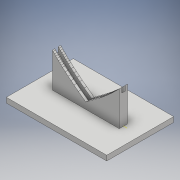
# Autodesk Inventor part: Supporto2
Saved by Autodesk Inventor 2018 (Build 220112000, 112)
## iProperties
Created: 2020-01-19
Part Number: Supporto2
Material: Generic
Document SubType Name: Modeling
Designer: Lorenzo Spadaro
Density: 1 g/cm^3
Appearance: Default
Author: Lorenzo Spadaro
Autodesk Inventor part; units mm, degrees
ref_plane "YZ Plane" through (0, 0, 0) normal (1, 0, 0) x (0, 1, 0)
ref_plane "XZ Plane" through (0, 0, 0) normal (0, 1, 0) x (-1, 0, 0)
ref_plane "XY Plane" through (0, 0, 0) normal (0, 0, 1) x (1, 0, 0)
sketch "Sketch1" plane through (0, 0, 0) normal (0, 0, 1) x (1, 0, 0)
  line L0 (-20, -20) -> (20, -20)
  line L1 (20, -20) -> (20, 20)
  line L2 (20, 20) -> (-20, 20)
  line L3 (-20, 20) -> (-20, -20)
  line L4 (-20, -20) -> (20, 20) construction
  line L5 (20, -20) -> (-20, 20) construction
  point P0 (0, 0)
  dimension "d0" = 40
  dimension "d1" = 40
  constraints: 12 end point, 2 midpoint, 2 parallel, 1 horizontal, 1 perpendicular
  measures "d0" distance of L2.end L1.end
  measures "d1" distance of L1.end L0.end
extrude "Extrusion1" add sketch "Sketch1" along normal blind 3
ref_plane "Work Plane1" through (-20, 0, 0) normal (0, -1, 0) x (1, 0, 0)
sketch "Sketch2" plane through (-20, 0, 0) normal (0, -1, 0) x (1, 0, 0)
  line L0 (0, 3) -> (40, 3)
  line L1 (0, 3) -> (40, 3) projected
  line L2 (2.7399, 64.6358) -> (3.1064, 64.6633)
  line L3 (3.1064, 64.6633) -> (5.3254, 64.7366)
  line L4 (5.3254, 64.7366) -> (6.8098, 64.6805)
  line L5 (6.8098, 64.6805) -> (7.9171, 64.5726)
  line L6 (7.9171, 64.5726) -> (9.0137, 64.4014)
  line L7 (9.0137, 64.4014) -> (9.7363, 64.2487)
  line L8 (9.7363, 64.2487) -> (10.4503, 64.0633)
  line L9 (10.4503, 64.0633) -> (11.1543, 63.8429)
  line L10 (11.1543, 63.8429) -> (11.8466, 63.5859)
  line L11 (11.8466, 63.5859) -> (12.5259, 63.2902)
  line L12 (12.5259, 63.2902) -> (13.1906, 62.9542)
  line L13 (13.1906, 62.9542) -> (13.4715, 62.803)
  line L14 (13.4715, 62.803) -> (14.2878, 62.3129)
  line L15 (14.2878, 62.3129) -> (15.32, 61.5828)
  line L16 (15.32, 61.5828) -> (16.5315, 60.5677)
  line L17 (16.5315, 60.5677) -> (20.0008, 56.8714)
  line L18 (20.0008, 56.8714) -> (23.8357, 60.8912)
  line L19 (23.8357, 60.8912) -> (25.2129, 61.9747)
  line L20 (25.2129, 61.9747) -> (26.196, 62.6151)
  line L21 (26.196, 62.6151) -> (26.5392, 62.8162)
  line L22 (26.5392, 62.8162) -> (26.8872, 63.0056)
  line L23 (26.8872, 63.0056) -> (27.2398, 63.1837)
  line L24 (27.2398, 63.1837) -> (27.5967, 63.3505)
  line L25 (27.5967, 63.3505) -> (27.9576, 63.5065)
  line L26 (27.9576, 63.5065) -> (28.6909, 63.787)
  line L27 (28.6909, 63.787) -> (29.4377, 64.0268)
  line L28 (29.4377, 64.0268) -> (30.1962, 64.2283)
  line L29 (30.1962, 64.2283) -> (30.9647, 64.3931)
  line L30 (30.9647, 64.3931) -> (31.7412, 64.5234)
  line L31 (31.7412, 64.5234) -> (32.5239, 64.6211)
  line L32 (32.5239, 64.6211) -> (33.7056, 64.711)
  line L33 (33.7056, 64.711) -> (35.2857, 64.7355)
  line L34 (35.2857, 64.7355) -> (37.2476, 64.6353)
  line L35 (37.2476, 64.6353) -> (37.63, 64.5998)
  line L36 (37.63, 64.5998) -> (38.0105, 64.5528)
  line L37 (38.0105, 64.5528) -> (38.3888, 64.4946)
  line L38 (38.3888, 64.4946) -> (39.1384, 64.3456)
  line L39 (39.1384, 64.3456) -> (39.8773, 64.1541)
  line L40 (39.8773, 64.1541) -> (40.6042, 63.922)
  line L41 (40.6042, 63.922) -> (41.3175, 63.6507)
  line L42 (41.3175, 63.6507) -> (42.016, 63.342)
  line L43 (42.016, 63.342) -> (42.6982, 62.9974)
  line L44 (42.6982, 62.9974) -> (43.3626, 62.6184)
  line L45 (43.3626, 62.6184) -> (44.0079, 62.2069)
  line L46 (44.0079, 62.2069) -> (44.6325, 61.7642)
  line L47 (44.6325, 61.7642) -> (45.2352, 61.2922)
  line L48 (45.2352, 61.2922) -> (45.8145, 60.7922)
  line L49 (45.8145, 60.7922) -> (46.3689, 60.2662)
  line L50 (46.3689, 60.2662) -> (46.8971, 59.7155)
  line L51 (46.8971, 59.7155) -> (47.2127, 59.3682)
  line L52 (47.2127, 59.3682) -> (47.5175, 59.0127)
  line L53 (47.5175, 59.0127) -> (47.8117, 58.6495)
  line L54 (47.8117, 58.6495) -> (48.0953, 58.2789)
  line L55 (48.0953, 58.2789) -> (48.3683, 57.901)
  line L56 (48.3683, 57.901) -> (48.631, 57.5163)
  line L57 (48.631, 57.5163) -> (48.8832, 57.1249)
  line L58 (48.8832, 57.1249) -> (49.1252, 56.7273)
  line L59 (49.1252, 56.7273) -> (49.3571, 56.3236)
  line L60 (49.3571, 56.3236) -> (49.5788, 55.9142)
  line L61 (49.5788, 55.9142) -> (49.7904, 55.4993)
  line L62 (49.7904, 55.4993) -> (50.1842, 54.6545)
  line L63 (50.1842, 54.6545) -> (50.5388, 53.7914)
  line L64 (50.5388, 53.7914) -> (50.8551, 52.9125)
  line L65 (50.8551, 52.9125) -> (51.1337, 52.02)
  line L66 (51.1337, 52.02) -> (51.3753, 51.1164)
  line L67 (51.3753, 51.1164) -> (51.5805, 50.2039)
  line L68 (51.5805, 50.2039) -> (51.75, 49.285)
  line L69 (51.75, 49.285) -> (51.8844, 48.3619)
  line L70 (51.8844, 48.3619) -> (51.9845, 47.437)
  line L71 (51.9845, 47.437) -> (51.9845, 43.3851)
  line L72 (51.9845, 43.3851) -> (51.9243, 42.8006)
  line L73 (51.9243, 42.8006) -> (51.8499, 42.2155)
  line L74 (51.8499, 42.2155) -> (51.7619, 41.6333)
  line L75 (51.7619, 41.6333) -> (51.6607, 41.054)
  line L76 (51.6607, 41.054) -> (51.5466, 40.4777)
  line L77 (51.5466, 40.4777) -> (51.4199, 39.9045)
  line L78 (51.4199, 39.9045) -> (51.2809, 39.3344)
  line L79 (51.2809, 39.3344) -> (51.13, 38.7676)
  line L80 (51.13, 38.7676) -> (50.9673, 38.204)
  line L81 (50.9673, 38.204) -> (50.7934, 37.6437)
  line L82 (50.7934, 37.6437) -> (50.6084, 37.0868)
  line L83 (50.6084, 37.0868) -> (50.2065, 35.9835)
  line L84 (50.2065, 35.9835) -> (49.7643, 34.8947)
  line L85 (49.7643, 34.8947) -> (49.2842, 33.8209)
  line L86 (49.2842, 33.8209) -> (48.7687, 32.7625)
  line L87 (48.7687, 32.7625) -> (48.2203, 31.7202)
  line L88 (48.2203, 31.7202) -> (47.6416, 30.6945)
  line L89 (47.6416, 30.6945) -> (46.7221, 29.1882)
  line L90 (46.7221, 29.1882) -> (45.7483, 27.7223)
  line L91 (45.7483, 27.7223) -> (45.2527, 27.0233)
  line L92 (45.2527, 27.0233) -> (44.7473, 26.3323)
  line L93 (44.7473, 26.3323) -> (44.2325, 25.649)
  line L94 (44.2325, 25.649) -> (43.7084, 24.9733)
  line L95 (43.7084, 24.9733) -> (43.1754, 24.305)
  line L96 (43.1754, 24.305) -> (42.0839, 22.9901)
  line L97 (42.0839, 22.9901) -> (40.96, 21.703)
  line L98 (40.96, 21.703) -> (39.806, 20.4424)
  line L99 (39.806, 20.4424) -> (38.6242, 19.2071)
  line L100 (38.6242, 19.2071) -> (37.4168, 17.9958)
  line L101 (37.4168, 17.9958) -> (35.5626, 16.2211)
  line L102 (35.5626, 16.2211) -> (33.6634, 14.4931)
  line L103 (33.6634, 14.4931) -> (30.4186, 11.7057)
  line L104 (30.4186, 11.7057) -> (28.4362, 10.0816)
  line L105 (28.4362, 10.0816) -> (20.0016, 3.7839)
  line L106 (20.0016, 3.7839) -> (15.5199, 7.0446)
  line L107 (15.5199, 7.0446) -> (12.8715, 9.064)
  line L108 (12.8715, 9.064) -> (11.1293, 10.4411)
  line L109 (11.1293, 10.4411) -> (9.4094, 11.8452)
  line L110 (9.4094, 11.8452) -> (7.7149, 13.2787)
  line L111 (7.7149, 13.2787) -> (6.0489, 14.7435)
  line L112 (6.0489, 14.7435) -> (5.2275, 15.4884)
  line L113 (5.2275, 15.4884) -> (4.4145, 16.242)
  line L114 (4.4145, 16.242) -> (3.6101, 17.0045)
  line L115 (3.6101, 17.0045) -> (2.8148, 17.7762)
  line L116 (2.8148, 17.7762) -> (2.0289, 18.5574)
  line L117 (2.0289, 18.5574) -> (1.2528, 19.3484)
  line L118 (1.2528, 19.3484) -> (0.487, 20.1494)
  line L119 (0.487, 20.1494) -> (-0.2682, 20.9606)
  line L120 (-0.2682, 20.9606) -> (-1.0124, 21.7824)
  line L121 (-1.0124, 21.7824) -> (-1.7452, 22.6151)
  line L122 (-1.7452, 22.6151) -> (-2.4663, 23.4588)
  line L123 (-2.4663, 23.4588) -> (-3.1752, 24.3139)
  line L124 (-3.1752, 24.3139) -> (-3.8715, 25.1807)
  line L125 (-3.8715, 25.1807) -> (-4.7177, 26.2914)
  line L126 (-4.7177, 26.2914) -> (-5.5375, 27.4273)
  line L127 (-5.5375, 27.4273) -> (-6.3273, 28.5876)
  line L128 (-6.3273, 28.5876) -> (-7.0831, 29.7717)
  line L129 (-7.0831, 29.7717) -> (-7.4472, 30.3726)
  line L130 (-7.4472, 30.3726) -> (-7.8013, 30.9792)
  line L131 (-7.8013, 30.9792) -> (-8.1451, 31.5915)
  line L132 (-8.1451, 31.5915) -> (-8.4779, 32.2094)
  line L133 (-8.4779, 32.2094) -> (-8.7995, 32.8328)
  line L134 (-8.7995, 32.8328) -> (-9.1093, 33.4617)
  line L135 (-9.1093, 33.4617) -> (-9.4067, 34.096)
  line L136 (-9.4067, 34.096) -> (-9.6915, 34.7356)
  line L137 (-9.6915, 34.7356) -> (-9.9629, 35.3804)
  line L138 (-9.9629, 35.3804) -> (-10.2207, 36.0305)
  line L139 (-10.2207, 36.0305) -> (-10.4643, 36.6856)
  line L140 (-10.4643, 36.6856) -> (-10.6932, 37.3458)
  line L141 (-10.6932, 37.3458) -> (-10.907, 38.0109)
  line L142 (-10.907, 38.0109) -> (-11.1052, 38.6809)
  line L143 (-11.1052, 38.6809) -> (-11.2872, 39.3557)
  line L144 (-11.2872, 39.3557) -> (-11.4527, 40.0352)
  line L145 (-11.4527, 40.0352) -> (-11.6012, 40.7195)
  line L146 (-11.6012, 40.7195) -> (-11.7322, 41.4083)
  line L147 (-11.7322, 41.4083) -> (-11.8451, 42.1017)
  line L148 (-11.8451, 42.1017) -> (-11.9396, 42.7995)
  line L149 (-11.9396, 42.7995) -> (-12.0151, 43.5017)
  line L150 (-12.0151, 43.5017) -> (-12.0151, 47.195)
  line L151 (-12.0151, 47.195) -> (-11.8821, 48.423)
  line L152 (-11.8821, 48.423) -> (-11.6913, 49.646)
  line L153 (-11.6913, 49.646) -> (-11.4406, 50.8589)
  line L154 (-11.4406, 50.8589) -> (-11.1277, 52.0567)
  line L155 (-11.1277, 52.0567) -> (-10.7505, 53.2347)
  line L156 (-10.7505, 53.2347) -> (-10.4622, 54.0065)
  line L157 (-10.4622, 54.0065) -> (-10.1438, 54.7658)
  line L158 (-10.1438, 54.7658) -> (-9.7945, 55.511)
  line L159 (-9.7945, 55.511) -> (-9.4137, 56.2409)
  line L160 (-9.4137, 56.2409) -> (-9.0008, 56.9538)
  line L161 (-9.0008, 56.9538) -> (-8.5551, 57.6483)
  line L162 (-8.5551, 57.6483) -> (-8.076, 58.323)
  line L163 (-8.076, 58.323) -> (-7.807, 58.6753)
  line L164 (-7.807, 58.6753) -> (-7.5285, 59.0209)
  line L165 (-7.5285, 59.0209) -> (-7.2406, 59.3595)
  line L166 (-7.2406, 59.3595) -> (-6.9435, 59.6908)
  line L167 (-6.9435, 59.6908) -> (-6.6375, 60.0145)
  line L168 (-6.6375, 60.0145) -> (-6.3229, 60.3303)
  line L169 (-6.3229, 60.3303) -> (-5.9999, 60.6377)
  line L170 (-5.9999, 60.6377) -> (-5.6688, 60.9366)
  line L171 (-5.6688, 60.9366) -> (-5.3297, 61.2265)
  line L172 (-5.3297, 61.2265) -> (-4.9829, 61.5071)
  line L173 (-4.9829, 61.5071) -> (-4.6287, 61.7781)
  line L174 (-4.6287, 61.7781) -> (-4.2674, 62.0391)
  line L175 (-4.2674, 62.0391) -> (-3.8989, 62.2899)
  line L176 (-3.8989, 62.2899) -> (-3.5239, 62.5301)
  line L177 (-3.5239, 62.5301) -> (-3.1425, 62.7594)
  line L178 (-3.1425, 62.7594) -> (-2.7548, 62.9773)
  line L179 (-2.7548, 62.9773) -> (-2.3611, 63.1837)
  line L180 (-2.3611, 63.1837) -> (-1.9617, 63.3782)
  line L181 (-1.9617, 63.3782) -> (-1.5569, 63.5603)
  line L182 (-1.5569, 63.5603) -> (-1.1468, 63.73)
  line L183 (-1.1468, 63.73) -> (-0.7316, 63.8867)
  line L184 (-0.7316, 63.8867) -> (-0.3117, 64.0302)
  line L185 (-0.3117, 64.0302) -> (0.1126, 64.16)
  line L186 (0.1126, 64.16) -> (0.5413, 64.276)
  line L187 (0.5413, 64.276) -> (0.9739, 64.3778)
  line L188 (0.9739, 64.3778) -> (1.4104, 64.465)
  line L189 (1.4104, 64.465) -> (1.8503, 64.5372)
  line L190 (1.8503, 64.5372) -> (2.2936, 64.5943)
  line L191 (2.2936, 64.5943) -> (2.7399, 64.6358)
  line L192 (0, 3) -> (0, 20.6726)
  line L193 (40, 0) -> (40, 3) projected
  line L194 (40, 3) -> (40, 20.6543)
  point P0 (20, 0)
  dimension "d0" = 40
  constraints: 386 end point, 4 perpendicular, 2 point on line, 1 collinear, 1 horizontal, 1 parallel
extrude "Extrusion2" add sketch "Sketch2" along normal mid plane 5 contours L192 L119 L118 L117 L116 L115 L114 L113 L112 L111 L110 L109 L108 L107 L106 L105 L104 L103 L102 L101 L100 L99 L98 L194 L0
sketch "Sketch3" plane through (0, 0, 3) normal (0, 0, 1) x (1, 0, 0)
  point P0 (0, 0)
sketch "Sketch4" plane through (-20, -2.5, 0) normal (0, -1, 0) x (1, 0, 0)
  line L0 (0.487, 20.1494) -> (0, 20.6726) projected
  line L1 (1.2528, 19.3484) -> (0.487, 20.1494) projected
  line L2 (2.0289, 18.5574) -> (1.2528, 19.3484) projected
  line L3 (2.8148, 17.7762) -> (2.0289, 18.5574) projected
  line L4 (3.6101, 17.0045) -> (2.8148, 17.7762) projected
  line L5 (4.4145, 16.242) -> (3.6101, 17.0045) projected
  line L6 (5.2275, 15.4884) -> (4.4145, 16.242) projected
  line L7 (6.0489, 14.7435) -> (5.2275, 15.4884) projected
  line L8 (7.7149, 13.2787) -> (6.0489, 14.7435) projected
  line L9 (9.4094, 11.8452) -> (7.7149, 13.2787) projected
  line L10 (11.1293, 10.4411) -> (9.4094, 11.8452) projected
  line L11 (12.8715, 9.064) -> (11.1293, 10.4411) projected
  line L12 (15.5199, 7.0446) -> (12.8715, 9.064) projected
  line L13 (40, 3) -> (0, 3) projected
  line L14 (40, 3) -> (40, 20.6543) projected
  line L15 (40, 20.6543) -> (39.806, 20.4424) projected
  line L16 (39.806, 20.4424) -> (38.6242, 19.2071) projected
  line L17 (38.6242, 19.2071) -> (37.4168, 17.9958) projected
  line L18 (37.4168, 17.9958) -> (35.5626, 16.2211) projected
  line L19 (35.5626, 16.2211) -> (33.6634, 14.4931) projected
  line L20 (33.6634, 14.4931) -> (30.4186, 11.7057) projected
  line L21 (30.4186, 11.7057) -> (28.4362, 10.0816) projected
  line L22 (28.4362, 10.0816) -> (20.0016, 3.7839) projected
  line L23 (20.0016, 3.7839) -> (15.5199, 7.0446) projected
  line L24 (15.5199, 7.0446) -> (12.8715, 9.064) projected
  line L25 (12.8715, 9.064) -> (11.1293, 10.4411) projected
  line L26 (11.1293, 10.4411) -> (9.4094, 11.8452) projected
  line L27 (9.4094, 11.8452) -> (7.7149, 13.2787) projected
  line L28 (7.7149, 13.2787) -> (6.0489, 14.7435) projected
  line L29 (6.0489, 14.7435) -> (5.2275, 15.4884) projected
  line L30 (5.2275, 15.4884) -> (4.4145, 16.242) projected
  line L31 (4.4145, 16.242) -> (3.6101, 17.0045) projected
  line L32 (3.6101, 17.0045) -> (2.8148, 17.7762) projected
  line L33 (2.8148, 17.7762) -> (2.0289, 18.5574) projected
  line L34 (2.0289, 18.5574) -> (1.2528, 19.3484) projected
  line L35 (1.2528, 19.3484) -> (0.487, 20.1494) projected
  line L36 (0.487, 20.1494) -> (0, 20.6726) projected
  line L37 (0, 20.6726) -> (0, 3) projected
  line L38 (28.4362, 10.0816) -> (20.0016, 3.7839) projected
  line L39 (20.0016, 3.7839) -> (40.0016, 3.7839) construction
  line L40 (0.487, 23.1494) -> (0, 23.6726)
  line L41 (1.2528, 22.3484) -> (0.487, 23.1494)
  line L42 (2.0289, 21.5574) -> (1.2528, 22.3484)
  line L43 (2.8148, 20.7762) -> (2.0289, 21.5574)
  line L44 (3.6101, 20.0045) -> (2.8148, 20.7762)
  line L45 (4.4145, 19.242) -> (3.6101, 20.0045)
  line L46 (5.2275, 18.4884) -> (4.4145, 19.242)
  line L47 (6.0489, 17.7435) -> (5.2275, 18.4884)
  line L48 (7.7149, 16.2787) -> (6.0489, 17.7435)
  line L49 (9.4094, 14.8452) -> (7.7149, 16.2787)
  line L50 (11.1293, 13.4411) -> (9.4094, 14.8452)
  line L51 (12.8715, 12.064) -> (11.1293, 13.4411)
  line L52 (15.5199, 10.0446) -> (12.8715, 12.064)
  line L53 (40, 23.6543) -> (39.806, 23.4424)
  line L54 (39.806, 23.4424) -> (38.6242, 22.2071)
  line L55 (38.6242, 22.2071) -> (37.4168, 20.9958)
  line L56 (37.4168, 20.9958) -> (35.5626, 19.2211)
  line L57 (35.5626, 19.2211) -> (33.6634, 17.4931)
  line L58 (33.6634, 17.4931) -> (30.4186, 14.7057)
  line L59 (30.4186, 14.7057) -> (28.4362, 13.0816)
  line L60 (28.4362, 13.0816) -> (20.0016, 6.7839)
  line L61 (20.0016, 6.7839) -> (15.5199, 10.0446)
  line L62 (15.5199, 10.0446) -> (12.8715, 12.064)
  line L63 (12.8715, 12.064) -> (11.1293, 13.4411)
  line L64 (11.1293, 13.4411) -> (9.4094, 14.8452)
  line L65 (9.4094, 14.8452) -> (7.7149, 16.2787)
  line L66 (7.7149, 16.2787) -> (6.0489, 17.7435)
  line L67 (6.0489, 17.7435) -> (5.2275, 18.4884)
  line L68 (5.2275, 18.4884) -> (4.4145, 19.242)
  line L69 (4.4145, 19.242) -> (3.6101, 20.0045)
  line L70 (3.6101, 20.0045) -> (2.8148, 20.7762)
  line L71 (2.8148, 20.7762) -> (2.0289, 21.5574)
  line L72 (2.0289, 21.5574) -> (1.2528, 22.3484)
  line L73 (1.2528, 22.3484) -> (0.487, 23.1494)
  line L74 (0.487, 23.1494) -> (0, 23.6726)
  line L75 (28.4362, 13.0816) -> (20.0016, 6.7839)
  line L76 (20.0016, 6.7839) -> (40.0016, 6.7839) construction
  line L77 (20.0016, 3.7839) -> (20.0016, 6.7839)
  line L78 (0, 23.6726) -> (0, 20.6726)
  line L79 (40, 23.6543) -> (40, 20.6543)
  point P0 (20, 0)
  dimension "d15" = 3
  constraints: 82 end point, 2 horizontal, 1 collinear, 1 parallel
  measures "d15" distance of L22.end L77.end
extrude "Extrusion3" add sketch "Sketch4" against normal blind 1.5 contours L0 L78 L40 L41 L42 L43 L44 L45 L46 L47 L48 L49 L50 L51 L52 L61 L77 L23 L12 L11 L10 L9 L8 L7 L6 L5 L4 L3 L2 L1 | L15 L16 L17 L18 L19 L20 L21 L22 L77 L60 L59 L58 L57 L56 L55 L54 L53 L79
sketch "Sketch5" plane through (-20, 2.5, 0) normal (0, 1, 0) x (1, 0, 0)
  line L0 (40, -23.6543) -> (40, -20.6543) projected
  line L1 (39.806, -20.4424) -> (40, -20.6543) projected
  line L2 (38.6242, -19.2071) -> (39.806, -20.4424) projected
  line L3 (37.4168, -17.9958) -> (38.6242, -19.2071) projected
  line L4 (35.5626, -16.2211) -> (37.4168, -17.9958) projected
  line L5 (33.6634, -14.4931) -> (35.5626, -16.2211) projected
  line L6 (30.4186, -11.7057) -> (33.6634, -14.4931) projected
  line L7 (28.4362, -10.0816) -> (30.4186, -11.7057) projected
  line L8 (20.0016, -3.7839) -> (28.4362, -10.0816) projected
  line L9 (15.5199, -7.0446) -> (20.0016, -3.7839) projected
  line L10 (12.8715, -9.064) -> (15.5199, -7.0446) projected
  line L11 (11.1293, -10.4411) -> (12.8715, -9.064) projected
  line L12 (9.4094, -11.8452) -> (11.1293, -10.4411) projected
  line L13 (7.7149, -13.2787) -> (9.4094, -11.8452) projected
  line L14 (6.0489, -14.7435) -> (7.7149, -13.2787) projected
  line L15 (5.2275, -15.4884) -> (6.0489, -14.7435) projected
  line L16 (4.4145, -16.242) -> (5.2275, -15.4884) projected
  line L17 (3.6101, -17.0045) -> (4.4145, -16.242) projected
  line L18 (2.8148, -17.7762) -> (3.6101, -17.0045) projected
  line L19 (2.0289, -18.5574) -> (2.8148, -17.7762) projected
  line L20 (1.2528, -19.3484) -> (2.0289, -18.5574) projected
  line L21 (0.487, -20.1494) -> (1.2528, -19.3484) projected
  line L22 (0, -20.6726) -> (0.487, -20.1494) projected
  line L23 (0, -20.6726) -> (0, -23.6726) projected
  line L24 (0, -23.6726) -> (0.487, -23.1494) projected
  line L25 (0.487, -23.1494) -> (1.2528, -22.3484) projected
  line L26 (1.2528, -22.3484) -> (2.0289, -21.5574) projected
  line L27 (2.0289, -21.5574) -> (2.8148, -20.7762) projected
  line L28 (2.8148, -20.7762) -> (3.6101, -20.0045) projected
  line L29 (3.6101, -20.0045) -> (4.4145, -19.242) projected
  line L30 (4.4145, -19.242) -> (5.2275, -18.4884) projected
  line L31 (5.2275, -18.4884) -> (6.0489, -17.7435) projected
  line L32 (6.0489, -17.7435) -> (7.7149, -16.2787) projected
  line L33 (7.7149, -16.2787) -> (9.4094, -14.8452) projected
  line L34 (9.4094, -14.8452) -> (11.1293, -13.4411) projected
  line L35 (11.1293, -13.4411) -> (12.8715, -12.064) projected
  line L36 (12.8715, -12.064) -> (15.5199, -10.0446) projected
  line L37 (15.5199, -10.0446) -> (20.0016, -6.7839) projected
  line L38 (20.0016, -6.7839) -> (28.4362, -13.0816) projected
  line L39 (28.4362, -13.0816) -> (30.4186, -14.7057) projected
  line L40 (30.4186, -14.7057) -> (33.6634, -17.4931) projected
  line L41 (33.6634, -17.4931) -> (35.5626, -19.2211) projected
  line L42 (35.5626, -19.2211) -> (37.4168, -20.9958) projected
  line L43 (37.4168, -20.9958) -> (38.6242, -22.2071) projected
  line L44 (38.6242, -22.2071) -> (39.806, -23.4424) projected
  line L45 (39.806, -23.4424) -> (40, -23.6543) projected
  point P0 (20, 0)
extrude "Extrusion4" add sketch "Sketch5" against normal blind 1.5
sketch "Sketch6" plane through (20, -20, 0) normal (1, 0, 0) x (0, 0, -1)
  line L0 (-3, 17.5) -> (-3, 0) projected
  line L1 (-3, 0) -> (-3, 40)
  line L2 (0, 40) -> (-3, 40) projected
  line L3 (-3, 40) -> (0, 40)
  line L4 (0, 40) -> (0, 0)
  line L5 (0, 0) -> (-3, 0)
  point P0 (0, 20)
  constraints: 8 end point, 3 perpendicular, 1 vertical
extrude "Extrusion5" add sketch "Sketch6" along normal blind 10
sketch "Sketch7" plane through (-20, -20, 0) normal (-1, 0, 0) x (0, 0, 1)
  line L0 (0, 40) -> (3, 40) projected
  line L1 (3, 17.5) -> (3, 0) projected
  line L2 (3, 40) -> (3, 0)
  line L3 (0, 0) -> (3, 0) projected
  line L4 (3, 0) -> (0, 0)
  line L5 (0, 0) -> (0, 40)
  line L6 (0, 40) -> (3, 40)
  point P0 (0, 20)
  constraints: 8 end point, 2 perpendicular, 1 collinear, 1 vertical
extrude "Extrusion6" add sketch "Sketch7" along normal blind 10
body "Solid1"
